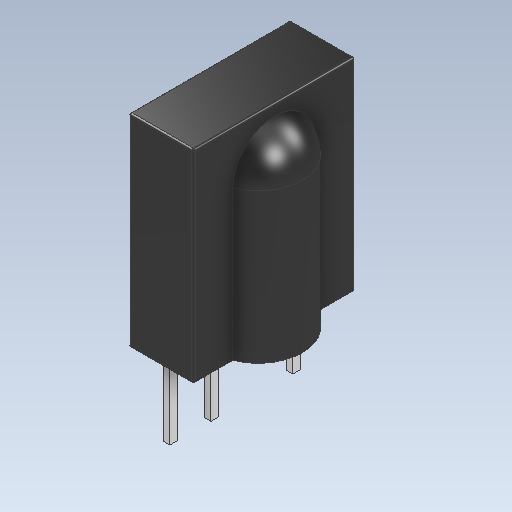
# Autodesk Inventor part: TSOP312
Saved by Autodesk Inventor 2020 (Build 240168000, 168)
## iProperties
Created: 2019-12-28
Part Number: TSOP312
Material: Generic
Document SubType Name: Modeling
Designer: ermoz
Density: 1 g/cm^3
Appearance: Default
Mass: 0.573841 g
Surface Area: 4.77805 cm^2
Volume: 0.573841 cm^3
Author: ermoz
Autodesk Inventor part; units mm, degrees
ref_plane "YZ Plane" through (0, 0, 0) normal (1, 0, 0) x (0, 1, 0)
ref_plane "XZ Plane" through (0, 0, 0) normal (0, 1, 0) x (-1, 0, 0)
ref_plane "XY Plane" through (0, 0, 0) normal (0, 0, 1) x (1, 0, 0)
sketch "Sketch4" plane through (0, 0, 0) normal (1, 0, 0) x (0, 1, 0)
  line L0 (0, 0) -> (12, 0)
  line L1 (12, 0) -> (12, -2.75)
  line L2 (12, -2.75) -> (0, -2.75)
  line L3 (0, -2.75) -> (0, 0)
  line L4 (12, 0) -> (0, 0)
  line L5 (0, 0) -> (0, 2.75)
  line L6 (0, 2.75) -> (12, 2.75)
  line L7 (12, 2.75) -> (12, 0)
  circle A0 centre (9.25, 0) radius 2.75
  point P0 (9.25, 2.75)
  dimension "d7" = 12
  dimension "d8" = 2.75
  dimension "d9" = 12
  dimension "d10" = 2.75
  constraints: 16 end point, 4 parallel, 3 tangent, 2 horizontal, 2 perpendicular, 1 centre point
  measures "d7" distance of L1.end L2.end
  measures "d8" distance of L0.end L1.end
  measures "d9" distance of L5.end L6.end
  measures "d10" distance of L4.end L5.end
revolve "Revolution1" add sketch "Sketch4" angle 360 about axis through (0, 0, 0) along (0, 1, 0) picked at (9.8215, 0.7167) contours L5 L6 A0 L0 | A0 L0
sketch "Sketch5" plane through (0, 0, 0) normal (0, -1, 0) x (1, 0, 0)
  circle A0 centre (0, 0) radius 2.75 projected
  line L0 (0, 0) -> (1, 0)
  line L1 (1, 0) -> (1, 5)
  line L2 (1, 5) -> (-3, 5)
  line L3 (-3, 5) -> (-3, -5)
  line L4 (-3, -5) -> (1, -5)
  line L5 (1, -5) -> (1, 5)
  dimension "d12" = 1
  dimension "d13" = 5
  dimension "d14" = 4
  dimension "d15" = 10
  constraints: 12 end point, 2 horizontal, 2 parallel, 1 perpendicular, 1 vertical
  measures "d12" distance of L0.start L0.end
  measures "d13" distance of L0.end L1.end
  measures "d14" distance of L4.end L3.end
  measures "d15" distance of L3.end L2.end
extrude "Extrusion3" add sketch "Sketch5" against normal blind 12.5 contours L1 L5 A0 | A0 L5 L4 L3 L2 L1 picked at (-1.4731, -0.2204)
fillet "Fillet1" radius 0.1 8 edges at (1, 6.25, 5) (1, 12.5, 0) (-1, 12.5, 5) (-3, 12.5, 0) (1, 6.25, -5) (-1, 12.5, -5) (-3, 6.25, -5) (-3, 6.25, 5)
sketch "Sketch6" plane through (0, 0, 0) normal (0, -1, 0) x (1, 0, 0)
  line L0 (-3, -4.9) -> (-3, 4.9) projected
  line L1 (-1.8, 4.06) -> (-1.4, 4.06)
  line L2 (-1.4, 4.06) -> (-1.4, 3.56)
  line L3 (-1.4, 3.56) -> (-1.8, 3.56)
  line L4 (-1.8, 3.56) -> (-1.8, 4.06)
  line L5 (-1.8, 4.06) -> (-1.4, 3.56) construction
  line L6 (-1.4, 4.06) -> (-1.8, 3.56) construction
  line L7 (-1.8, -3.56) -> (-1.4, -3.56)
  line L8 (-1.4, -3.56) -> (-1.4, -4.06)
  line L9 (-1.4, -4.06) -> (-1.8, -4.06)
  line L10 (-1.8, -4.06) -> (-1.8, -3.56)
  line L11 (-1.8, -3.56) -> (-1.4, -4.06) construction
  line L12 (-1.4, -3.56) -> (-1.8, -4.06) construction
  line L13 (-1.8, 1.52) -> (-1.4, 1.52)
  line L14 (-1.4, 1.52) -> (-1.4, 1.02)
  line L15 (-1.4, 1.02) -> (-1.8, 1.02)
  line L16 (-1.8, 1.02) -> (-1.8, 1.52)
  line L17 (-1.8, 1.52) -> (-1.4, 1.02) construction
  line L18 (-1.4, 1.52) -> (-1.8, 1.02) construction
  point P0 (0, 0)
  dimension "d22" = 0.4
  dimension "d23" = 0.5
  dimension "d24" = 0.4
  dimension "d25" = 0.5
  dimension "d27" = 0.4
  dimension "d28" = 0.5
  constraints: 36 end point, 6 parallel, 3 horizontal, 3 perpendicular
  measures "d22" distance of L2.end L3.end
  measures "d23" distance of L1.end L2.end
  measures "d24" distance of L8.end L9.end
  measures "d25" distance of L7.end L8.end
  measures "d27" distance of L14.end L15.end
  measures "d28" distance of L13.end L14.end
extrude "Extrusion4" add sketch "Sketch6" along normal blind 5
fillet "Fillet2" radius 0.5 12 edges at (-1.8, 0, 3.81) (-1.6, 0, 4.06) (-1.4, 0, 3.81) (-1.6, 0, 3.56) (-1.4, 0, 1.27) (-1.6, 0, 1.52) (-1.8, 0, 1.27) (-1.6, 0, 1.02) (-1.8, 0, -3.81) (-1.6, 0, -4.06) (-1.4, 0, -3.81) (-1.6, 0, -3.56)
body "Solid2"
